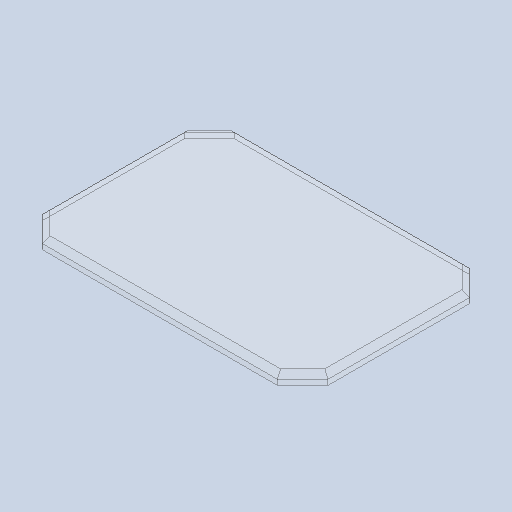
# Autodesk Inventor part: BigContainerLid
Saved by Autodesk Inventor 2024 (Build 280153000, 153)
## iProperties
Created: 2023-06-12
Part Number: BigContainerLid
Material: Polycarbonate, Clear
Document SubType Name: Modeling
Designer: 18179
Density: 1.2 g/cm^3
Appearance: Clear - Light
Author: 18179
Autodesk Inventor part; units mm, degrees
ref_plane "YZ Plane" through (0, 0, 0) normal (1, 0, 0) x (0, 1, 0)
ref_plane "XZ Plane" through (0, 0, 0) normal (0, 1, 0) x (-1, 0, 0)
ref_plane "XY Plane" through (0, 0, 0) normal (0, 0, 1) x (1, 0, 0)
sketch "Sketch3" plane through (0, 0, 0) normal (0, 1, 0) x (-1, 0, 0)
  line L0 (-344.5001, 169.0756) -> (-344.5001, -169.7218)
  line L1 (-344.5001, -169.7218) -> (-284.0287, -230.1931)
  line L2 (-284.0287, -230.1931) -> (278.2886, -230.1931)
  line L3 (278.2886, -230.1931) -> (338.7599, -169.7218)
  line L4 (338.7599, -169.7218) -> (338.7599, 169.0756)
  line L5 (338.7599, 169.0756) -> (278.2886, 229.5469)
  line L6 (278.2886, 229.5469) -> (-284.0287, 229.5469)
  line L7 (-284.0287, 229.5469) -> (-344.5001, 169.0756)
  line L8 (-278.7682, 216.8469) -> (-331.8001, 163.8151)
  line L9 (273.0281, 216.8469) -> (-278.7682, 216.8469)
  line L10 (326.0599, 163.8151) -> (273.0281, 216.8469)
  line L11 (326.0599, -164.4613) -> (326.0599, 163.8151)
  line L12 (273.0281, -217.4931) -> (326.0599, -164.4613)
  line L13 (-278.7682, -217.4931) -> (273.0281, -217.4931)
  line L14 (-331.8001, -164.4613) -> (-278.7682, -217.4931)
  line L15 (-331.8001, 163.8151) -> (-331.8001, -164.4613)
  point P0 (0, 0)
  point P1 (-344.5001, -230.1931)
  constraints: 32 end point
extrude "Extrusion3" add sketch "Sketch3" against normal blind 25.4 contours L7 L6 L5 L4 L3 L2 L1 L0 | L9 L10 L11 L12 L13 L14 L15 L8
chamfer "Chamfer1" distance 12.7 angle 45 8 edges at (-338.7599, 0, -0.3231) (-308.5243, 0, -199.9575) (2.8701, 0, -230.1931) (314.2644, 0, -199.9575) (344.5001, 0, -0.3231) (314.2644, 0, 199.3112) (2.8701, 0, 229.5469) (-308.5243, 0, 199.3112)
body "Solid2"
